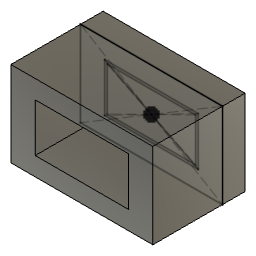
ChargePortMale v3 (Autodesk Fusion 360 archive; units mm, degrees)
design "AndersonPairHolderV1"
Autodesk Fusion 360 part; units mm, degrees
sketch "Sketch1" plane through (0, 0, 0) normal (0, 1, 0) x (1, 0, 0)
  line L0 (7.8, -3.815) -> (-7.8, -3.815)
  line L1 (-7.8, -3.815) -> (-7.8, 3.815)
  line L2 (-7.8, 3.815) -> (7.8, 3.815)
  line L3 (7.8, 3.815) -> (7.8, -3.815)
  line L4 (7.8, -3.815) -> (-7.8, 3.815) construction
  line L5 (-7.8, -3.815) -> (7.8, 3.815) construction
  line L6 (8.225, -4.25) -> (-8.225, -4.25)
  line L7 (-8.225, -4.25) -> (-8.225, 4.25)
  line L8 (-8.225, 4.25) -> (8.225, 4.25)
  line L9 (8.225, 4.25) -> (8.225, -4.25)
  line L10 (8.225, -4.25) -> (-8.225, 4.25) construction
  line L11 (-8.225, -4.25) -> (8.225, 4.25)
  line L12 (12.5, -7.5) -> (-12.5, -7.5)
  line L13 (-12.5, -7.5) -> (-12.5, 7.5)
  line L14 (-12.5, 7.5) -> (12.5, 7.5)
  line L15 (12.5, 7.5) -> (12.5, -7.5)
  line L16 (12.5, -7.5) -> (-12.5, 7.5) construction
  line L17 (-12.5, -7.5) -> (12.5, 7.5) construction
  dimension "d1" = 15.6
  dimension "d2" = 7.63
  dimension "d3" = 16.45
  dimension "d4" = 8.5
  dimension "d5" = 25
  dimension "d6" = 15
  constraint horizontal L0
  constraint perpendicular L0 L1
  constraint parallel L0 L2
  constraint parallel L1 L3
  constraint coincident L4 origin
  constraint coincident L5 origin
  constraint horizontal L6
  constraint perpendicular L6 L7
  constraint parallel L6 L8
  constraint parallel L7 L9
  constraint coincident L10 origin
  constraint coincident L11 origin
  constraint horizontal L12
  constraint perpendicular L12 L13
  constraint parallel L12 L14
  constraint parallel L13 L15
  constraint coincident L16 origin
  constraint coincident L17 origin
  measures "d1" distance of L1.end L2.end
  measures "d2" distance of L0.end L1.end
  measures "d3" distance of L7.end L8.end
  measures "d4" distance of L6.end L7.end
  measures "d5" distance of L13.end L14.end
  measures "d6" distance of L12.end L13.end
extrude "Extrude1" add sketch "Sketch1" against normal blind 12.25 makes body 1
extrude "Extrude2" add sketch "Sketch1" along normal blind 4 contours L0 L2 L3 L6 L9 L11 | L0 L1 L2 L7 L8 L11 | L12 L13 L14 L15 bodies 1
copy_body "Body->Comp1" bodies 1 removing the originals makes body 2 in component "PairHolder"
component "PairHolder" placed x (1, 0, 0) y (0, 1, 0) z (0, 0, 1) at (0, 0, 0)
